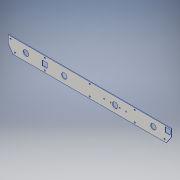
# Autodesk Inventor part: InsidePlate
Saved by Autodesk Inventor 2016 (Build 200138000, 138)
## iProperties
Created: 2017-01-19
Part Number: InsidePlate
Material: Aluminum 6061
Document SubType Name: Modeling
Designer: Kyle
Density: 2.7 g/cm^3
Appearance: Aluminum - Flat
Mass: 510.361 g
Surface Area: 1274.83 cm^2
Volume: 189.022 cm^3
Author: Kyle
Autodesk Inventor part; units mm, degrees
ref_plane "YZ Plane" through (0, 0, 0) normal (1, 0, 0) x (0, 1, 0)
ref_plane "XZ Plane" through (0, 0, 0) normal (0, 1, 0) x (-1, 0, 0)
ref_plane "XY Plane" through (0, 0, 0) normal (0, 0, 1) x (1, 0, 0)
sketch "Sketch1" plane through (0, 0, 0) normal (0, 0, 1) x (1, 0, 0)
  line L0 (0, 0) -> (850.9, 0)
  line L1 (850.9, 0) -> (850.9, 76.2)
  line L2 (850.9, 76.2) -> (0, 76.2)
  line L3 (0, 76.2) -> (0, 0)
  dimension "d0" = 850.9
  dimension "d1" = 76.2
  constraints: 8 end point, 2 parallel, 1 horizontal, 1 perpendicular
  measures "d0" distance of L2.end L1.end
  measures "d1" distance of L1.end L0.end
extrude "Extrusion1" add sketch "Sketch1" along normal blind 3.175
sketch "Sketch2" plane through (0, 0, 3.175) normal (0, 0, 1) x (1, 0, 0)
  line L0 (0, 0) -> (850.9, 0) projected
  circle A0 centre (292.9509, 36.5125) radius 14.2875
  circle A1 centre (557.9491, 36.5125) radius 14.2875
  circle A2 centre (92.9313, 39.6875) radius 14.2875
  circle A3 centre (757.9235, 39.6875) radius 14.2875
  line L1 (0, 0) -> (25.4, 0)
  line L2 (0, 0) -> (0, 38.1)
  line L3 (0, 76.2) -> (0, 0) projected
  line L4 (0, 38.1) -> (25.4, 0)
  circle A4 centre (34.925, 12.7) radius 3.5687
  circle A5 centre (12.7, 63.5) radius 3.5687
  line L5 (850.9, 76.2) -> (0, 76.2) projected
  line L6 (850.9, 0) -> (850.9, 38.1)
  line L7 (850.9, 0) -> (850.9, 76.2) projected
  line L8 (850.9, 0) -> (825.5, 0)
  line L9 (825.5, 0) -> (850.9, 38.1)
  circle A6 centre (190.5, 38.1) radius 3.5687
  line L10 (825.5, 0) -> (800.1, 0)
  circle A7 centre (815.975, 12.7) radius 3.5687
  circle A8 centre (831.85, 57.15) radius 3.5687
  circle A9 centre (425.45, 66.675) radius 3.5687
  circle A10 centre (425.45, 9.525) radius 3.5687
  circle A11 centre (190.5, 9.525) radius 3.5687
  circle A12 centre (190.5, 66.675) radius 3.5687
  circle A13 centre (660.4, 66.675) radius 3.5687
  circle A14 centre (660.4, 9.525) radius 3.5687
  dimension "d10" = 28.575
  dimension "d23" = 28.575
  dimension "d30" = 28.575
  dimension "d32" = 28.575
  dimension "d34" = 25.4
  dimension "d35" = 38.1
  dimension "d36" = 7.1374
  dimension "d37" = 12.7
  dimension "d38" = 9.525
  dimension "d40" = 7.1374
  dimension "d41" = 12.7
  dimension "d43" = 38.1
  dimension "d44" = 25.4
  dimension "d53" = 7.1374
  dimension "d54" = 38.1
  dimension "d55" = 190.5
  dimension "d59" = 7.1374
  dimension "d60" = 12.7
  dimension "d61" = 9.525
  dimension "d66" = 7.1374
  dimension "d67" = 7.1374
  dimension "d68" = 9.525
  dimension "d69" = 425.45
  dimension "d70" = 7.1374
  dimension "d71" = 9.525
  dimension "d72" = 425.45
  dimension "d73" = 7.1374
  dimension "d74" = 7.1374
  dimension "d75" = 9.525
  dimension "d76" = 9.525
  dimension "d77" = 190.5
  dimension "d78" = 190.5
  dimension "d79" = 7.1374
  dimension "d80" = 7.1374
  dimension "d81" = 9.525
  dimension "d82" = 9.525
  dimension "d83" = 190.5
  dimension "d84" = 190.5
  dimension "d103" = 12.7
  constraints: 15 centre point, 14 end point, 2 midpoint, 2 point on line, 1 horizontal
  measures "d10" diameter of A0
  measures "d23" diameter of A1
  measures "d30" diameter of A2
  measures "d32" diameter of A3
  measures "d34" distance of L0.start L1.end
  measures "d35" distance of L0.start L2.end
  measures "d36" diameter of A4
  measures "d37" distance from line of L0 A4.centre
  measures "d38" horizontal distance of L1.end A4.centre
  measures "d40" diameter of A5
  measures "d41" distance from line of L3 A5.centre
  measures "d43" distance of L0.end L6.end
  measures "d44" distance of L0.end L8.end
  measures "d53" diameter of A6
  measures "d54" distance from line of L0 A6.centre
  measures "d55" distance from line of L3 A6.centre
  measures "d59" diameter of A7
  measures "d60" distance from line of L0 A7.centre
  measures "d61" horizontal distance of L8.end A7.centre
  measures "d66" diameter of A8
  measures "d67" diameter of A9
  measures "d68" distance from line of L5 A9.centre
  measures "d69" distance from line of L3 A9.centre
  measures "d70" diameter of A10
  measures "d71" distance from line of L0 A10.centre
  measures "d72" distance from line of L3 A10.centre
  measures "d73" diameter of A11
  measures "d74" diameter of A12
  measures "d75" distance from line of L5 A12.centre
  measures "d76" distance from line of L0 A11.centre
  measures "d77" distance from line of L3 A12.centre
  measures "d78" distance from line of L2 A11.centre
  measures "d79" diameter of A13
  measures "d80" diameter of A14
  measures "d81" distance from line of L0 A14.centre
  measures "d82" distance from line of L5 A13.centre
  measures "d83" distance from line of L7 A13.centre
  measures "d84" distance from line of L6 A14.centre
  measures "d103" distance from line of L5 A5.centre
sketch "Sketch3" plane through (0, 0, 3.175) normal (0, 0, 1) x (1, 0, 0)
  circle A0 centre (190.5, 38.1) radius 3.5687 projected
  circle A1 centre (831.85, 57.15) radius 3.5687 projected
  line L0 (179.2605, 25.273) -> (201.7395, 25.273)
  line L1 (203.327, 26.8605) -> (203.327, 49.3395)
  line L2 (201.7395, 50.927) -> (179.2605, 50.927)
  line L3 (177.673, 49.3395) -> (177.673, 26.8605)
  line L4 (177.673, 25.273) -> (203.327, 50.927) construction
  line L5 (203.327, 25.273) -> (177.673, 50.927) construction
  line L6 (843.0895, 44.323) -> (820.6105, 44.323)
  line L7 (819.023, 45.9105) -> (819.023, 68.3895)
  line L8 (820.6105, 69.977) -> (843.0895, 69.977)
  line L9 (844.677, 68.3895) -> (844.677, 45.9105)
  line L10 (844.677, 44.323) -> (819.023, 69.977) construction
  line L11 (819.023, 44.323) -> (844.677, 69.977) construction
  circle A2 centre (581.7616, 36.5125) radius 2.8067
  circle A3 centre (534.1366, 36.5125) radius 2.8067
  circle A4 centre (500.7991, 36.5125) radius 2.8067
  circle A5 centre (615.0991, 36.5125) radius 2.8067
  arc A6 (179.2605, 50.927) -> (177.673, 49.3395) centre (179.2605, 49.3395) ccw
  arc A7 (203.327, 49.3395) -> (201.7395, 50.927) centre (201.7395, 49.3395) ccw
  arc A8 (201.7395, 25.273) -> (203.327, 26.8605) centre (201.7395, 26.8605) ccw
  arc A9 (177.673, 26.8605) -> (179.2605, 25.273) centre (179.2605, 26.8605) ccw
  arc A10 (820.6105, 69.977) -> (819.023, 68.3895) centre (820.6105, 68.3895) ccw
  arc A11 (844.677, 68.3895) -> (843.0895, 69.977) centre (843.0895, 68.3895) ccw
  arc A12 (843.0895, 44.323) -> (844.677, 45.9105) centre (843.0895, 45.9105) ccw
  arc A13 (819.023, 45.9105) -> (820.6105, 44.323) centre (820.6105, 45.9105) ccw
  point P0 (0, 0)
  dimension "d88" = 25.654
  dimension "d89" = 25.654
  dimension "d90" = 25.654
  dimension "d91" = 25.654
  dimension "d93" = 5.6134
  dimension "d94" = 5.6134
  dimension "d96" = 5.6134
  dimension "d97" = 5.6134
  dimension "d98" = 1.5875
  constraints: 24 end point, 16 point on circle, 16 point on line, 16 tangent, 12 centre point, 7 equal radius, 4 midpoint, 4 parallel, 2 horizontal, 2 perpendicular
  measures "d88" distance of L5.end L4.end
  measures "d89" distance of L4.end L5.start
  measures "d90" distance of L10.end L11.end
  measures "d91" distance of L11.start L10.end
  measures "d93" diameter of A2
  measures "d94" diameter of A3
  measures "d96" diameter of A4
  measures "d97" diameter of A5
  measures "d98" radius of A6
extrude "Extrusion4" cut sketch "Sketch3" against normal blind 25.4
extrude "Extrusion5" cut sketch "Sketch2" against normal blind 25.4 contours L2 L4 L0 | L9 L6 L0 | A0 | A1 | A2 | A3 | A4 | A5 | A6 | A7 | A8 | A9 | A10 | A11 | A12 | A13 | A14
body "Solid1"
